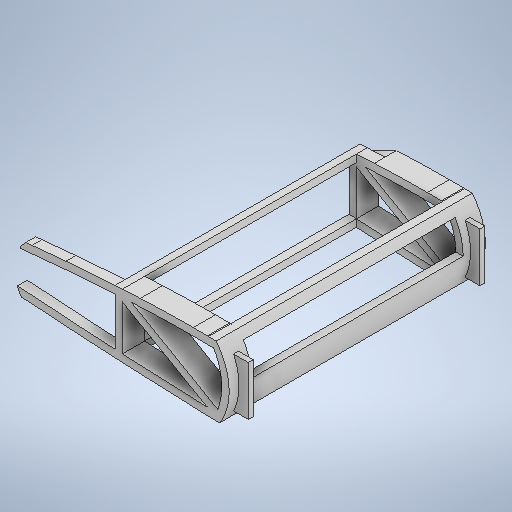
# Autodesk Inventor part: 1P.01.05.04-HB-PlatformFinala
Saved by Autodesk Inventor 2025.1 (Build 291241000, 241)
## iProperties
Created: 2025-01-16
Part Number: 1P.01.05.04-HB-PlatformFinala
Material: Generic
Document SubType Name: Modeling
Designer: hjbre
Density: 1 g/cm^3
Appearance: Default
Author: hjbre
Autodesk Inventor part; units mm, degrees
note: some values were not read from the file. Chosen so that the rebuilt part matches the saved one: second side of "Extrusion6".
ref_plane "YZ Plane" through (0, 0, 0) normal (1, 0, 0) x (0, 1, 0)
ref_plane "XZ Plane" through (0, 0, 0) normal (0, 1, 0) x (-1, 0, 0)
ref_plane "XY Plane" through (0, 0, 0) normal (0, 0, 1) x (1, 0, 0)
sketch "Sketch2" plane through (-116.745334, -43.168812, 0) normal (0, 0, 1) x (1, 0, 0)
  spline S0 degree 4 poles (254.436054, 38.258138) (252.159915, 38.650332) (246.788709, 39.499265) (237.984874, 40.618279) (225.357478, 41.704285) (211.202741, 42.341661) (196.392584, 42.47009) (181.031283, 42.070233) (165.506388, 41.221743) (149.785249, 40.04478) (134.1096, 38.577548) (118.624688, 36.850842) (103.500036, 34.939301) (88.901638, 32.883406) (74.995754, 30.738214) (61.917783, 28.562704) (49.827113, 26.40977) (38.835364, 24.340018) (29.07721, 22.403865) (20.632296, 20.65644) (13.645605, 19.149082) (6.913163, 17.660714) (2.90218, 16.740022) (0.469137, 16.188187) (0, 16.065) knots 0.21429705 0.21429705 0.21429705 0.21429705 0.21429705 0.2433201 0.28177524 0.32154178 0.36237973 0.40400459 0.44617789 0.48866482 0.5312306 0.57368816 0.61580317 0.65733642 0.6980466 0.73768213 0.77598623 0.81268845 0.84749504 0.88008735 0.91009265 0.93705903 0.9603631 1 1 1 1 1
  spline S1 degree 4 poles (299.999997, 15.624) (299.805651, 13.312974) (297.70854, 10.343184) (293.050897, 7.5008) (285.395888, 4.883043) (278.112378, 3.216454) (269.51472, 1.892454) (259.681019, 0.912997) (248.712883, 0.278332) (236.711867, -0.030891) (223.806667, -0.050368) (210.125319, 0.193333) (195.775416, 0.645033) (180.96771, 1.249367) (165.65166, 1.982539) (150.191633, 2.90484) (134.687258, 3.945111) (119.337536, 5.049498) (104.304233, 6.19869) (89.756609, 7.356132) (75.849243, 8.488651) (62.742937, 9.582405) (50.58108, 10.6226) (39.497058, 11.579661) (29.629443, 12.451258) (21.071102, 13.226419) (13.964229, 13.872003) (7.104281, 14.512735) (2.97189, 14.898983) (0.53364, 15.140199) (0, 15.183) knots 0 0 0 0 0 0.05437358 0.07982309 0.10791481 0.13850221 0.17134572 0.20619217 0.24278976 0.28089755 0.32028459 0.36072189 0.40203271 0.44399579 0.48638488 0.52897072 0.57147417 0.6136572 0.65528122 0.69610245 0.73587112 0.77432706 0.81119414 0.84617761 0.87895143 0.90913704 0.93627519 0.95973484 1 1 1 1 1
  arc A0 (0, 16.065) -> (0, 15.183) centre (0.115799, 15.624) ccw
  line L0 (0.115799, 15.624) -> (227.990221, 15.624) construction
  line L1 (299.999997, 15.624) -> (0.115799, 15.624) construction
  line L2 (299.999997, 15.624) -> (199.999997, 15.624) construction
  line L3 (199.999997, 15.624) -> (199.999997, 42.37734) construction
  line L4 (199.999997, 15.624) -> (199.999997, 0.52729)
  line L5 (0, 0) -> (0, 20.241)
  line L6 (0, 20.241) -> (238.581, 20.241) construction
  circle A1 centre (238.581, 20.241) radius 14
  line L7 (238.581, 20.241) -> (208.581, 20.241)
  line L8 (238.581, 25.359) -> (238.581, 20.241)
  line L9 (0, 20.241) -> (112, 20.241)
  circle A2 centre (112, 20.241) radius 5.39
  line L10 (0, 15.624) -> (112, 15.624) construction
  line L11 (0, 15.624) -> (112, 15.624) construction
  line L12 (112, 15.624) -> (112, 35.994456)
  line L13 (112, 15.624) -> (112, 5.61525)
  line L14 (299.207055, 20.082158) -> (298.87417, 19.536312) construction
  arc A3 (298.903999, 19.593162) -> (299.170168, 20.029611) centre (292.291091, 23.925437) ccw construction
  spline S2 degree 4 poles (299.285198, 20.241) (299.227939, 20.131643) (299.16804, 20.023225) (299.105573, 19.915754) (299.040612, 19.809235) knots 0 0 0 0 0 1 1 1 1 1
  line L15 (299.43203, 20.521431) -> (299.138367, 19.960569) construction
  arc A4 (299.163926, 20.01882) -> (299.398715, 20.467241) centre (292.801001, 23.636075) ccw construction
  line L16 (294.550692, 15.715716) -> (294.235931, 15.532284) construction
  arc A5 (294.267154, 15.551069) -> (294.518956, 15.69781) centre (283.884356, 33.65696) ccw construction
  spline S3 degree 2 poles (295.850621, 16.559978) (295.157262, 16.069203) (294.393311, 15.624) knots 0 0 0 1 1 1
  line L17 (295.959293, 16.465681) -> (295.74195, 16.654276) construction
  arc A6 (295.937354, 16.484307) -> (295.763482, 16.635181) centre (281.87292, 0.451609) ccw construction
  spline S4 degree 4 poles (296.856901, 15.624) (296.618326, 15.862944) (296.370731, 16.098547) (296.114674, 16.330852) (295.850621, 16.559978) knots 0 0 0 0 0 1 1 1 1 1
  spline S5 degree 4 poles (219.58717, 34.91187) (218.695351, 34.95198) (214.858509, 35.106335) (210.707211, 35.329502) (192.898023, 35.446366) (181.42777, 35.055508) (165.177387, 34.181901) (149.561876, 33.12667) (133.828431, 31.347909) (128.265438, 31.097419) (123.390775, 30.590026) knots 0 0 0 0 0 0.13924435 0.23321956 0.36393672 0.50998276 0.65711487 0.7981047 1 1 1 1 1
  line L18 (232.743774, 34.364452) -> (201.193566, 35.681454) construction
  arc A7 (229.586762, 34.454933) -> (204.347135, 35.508511) centre (136.348344, -1896.324468) ccw construction
  arc A8 (264.266057, 15.123) -> (264.360826, 15.624) centre (238.581, 20.241) ccw
  circle A9 centre (238.581, 20.241) radius 24
  circle A10 centre (112, 20.241) radius 15.39
  spline S6 degree 4 poles (299.999997, 15.624) (300.269142, 17.933652) (298.783415, 21.267693) (294.693448, 24.979847) (287.53174, 28.940551) (280.486947, 31.820538) (271.480983, 34.718213) (262.486804, 36.793013) (257.700386, 37.695672) (254.436054, 38.258138) knots 0 0 0 0 0 0.24755477 0.36385739 0.4925498 0.63299607 0.77826439 1 1 1 1 1
  line L19 (285.294543, 32.941011) -> (223.577565, 43.575266) construction
  arc A11 (278.722442, 32.634865) -> (229.668212, 41.087243) centre (217.218351, -177.738587) ccw construction
  line L20 (285.294543, 32.941011) -> (223.577565, 43.575266) construction
  arc A12 (278.877125, 33.041766) -> (229.658629, 41.522447) centre (200.894913, -272.473315) ccw construction
  line L21 (285.294543, 25.932171) -> (223.577565, 36.566425) construction
  spline S7 degree 4 poles (251.493, 31.73616) (243.700929, 32.967588) (232.160237, 34.296592) (216.442824, 35.287928) (196.392341, 35.461091) (181.031705, 35.061513) (165.505292, 34.212684) (149.788285, 33.036509) (134.101234, 31.567156) (118.647366, 29.846206) (103.439709, 27.919279) (89.058912, 25.903716) (74.837064, 23.692714) (62.488433, 21.669546) (49.639937, 19.354465) (46.379459, 18.742869) (43.812536, 18.259032) knots 0 0 0 0 0 0.1639631 0.23233838 0.3020312 0.37264227 0.44377843 0.51504665 0.58613365 0.65664712 0.72618654 0.7943479 0.86070997 0.92034602 1 1 1 1 1
  line L22 (285.294543, 25.932171) -> (223.577565, 36.566425) construction
  arc A13 (278.722442, 25.626025) -> (229.668212, 34.078402) centre (217.218351, -184.747428) ccw construction
  spline S8 degree 4 poles (295.845009, 16.556007) (295.719822, 16.664559) (294.584958, 17.628339) (292.058546, 19.428263) (287.516704, 21.93465) (280.467029, 24.832118) (271.97142, 27.522599) (264.208658, 29.400369) (258.409244, 30.551465) (255.053616, 31.142888) (254.436054, 31.249298) (253.968946, 31.329784) (253.501839, 31.41027) (253.034731, 31.490756) (252.567623, 31.571241) knots 0 0 0 0 0 0.01890503 0.16895946 0.33499927 0.51620401 0.71116085 0.9183366 0.96483207 0.96483207 0.96483207 0.96483207 1 1 1 1 1
  line L23 (270.129, 9.125374) -> (275.129, 9.125374) construction
  line L24 (281.07, 24.45816) -> (286.07, 24.45816) construction
  line L25 (318.821413, -3.367269) -> (272.868604, 36.479282) construction
  arc A14 (303.207925, 0.551953) -> (278.959518, 21.578206) centre (281.857648, 0.425162) ccw construction
  line L26 (68.488377, 16.119755) -> (19.136695, 20.398308) construction
  arc A15 (63.551474, 16.528056) -> (24.070206, 19.950891) centre (-819.899413, -9944.371227) ccw construction
  line L27 (21.724437, 20.217275) -> (21.200116, 20.264725) construction
  arc A16 (21.252548, 20.259982) -> (21.672005, 20.222022) centre (898.635849, 9712.955601) ccw construction
  spline S9 degree 4 poles (295.835285, 16.564433) (293.417091, 14.88464) (288.41352, 12.692641) (280.70627, 10.669821) (269.511023, 8.939829) (259.682627, 7.96324) (248.712204, 7.32734) (236.712148, 7.018633) (223.806545, 6.998947) (210.125394, 7.242728) (195.775305, 7.694406) (180.967993, 8.298721) (165.65086, 9.03198) (150.193891, 9.954022) (134.681006, 10.995018) (119.354518, 12.097424) (104.258979, 13.251926) (89.874814, 14.39542) (75.752353, 15.547068) (62.906491, 16.616479) (50.510696, 17.677636) (46.516568, 18.024605) (43.812536, 18.259032) knots 0 0 0 0 0 0.08476672 0.12402522 0.16617938 0.21090431 0.25787677 0.30678758 0.35734028 0.40924097 0.46226281 0.51612182 0.5705276 0.62518592 0.67973848 0.7338798 0.78730362 0.83969707 0.89073959 0.93714265 1 1 1 1 1
  spline S10 degree 4 poles (21.462276, 20.241) (20.622656, 20.316984) (20.124028, 20.362207) (19.919133, 20.380856) (19.554048, 20.414029) knots 0 0 0 0 0 1 1 1 1 1
  line L28 (74.254065, 23.996937) -> (13.371006, 12.521126) construction
  arc A17 (68.175943, 22.793945) -> (19.469999, 13.613391) centre (1053.390082, -5337.891027) ccw construction
  line L29 (133.533683, 10.96354) -> (115.839617, 12.094223) construction
  arc A18 (117.617989, 12.078874) -> (131.767822, 11.174674) centre (141.026952, 267.238396) ccw construction
  spline S11 degree 4 poles (218.437499, 7.193419) (217.617295, 7.240848) (213.819214, 7.468804) (209.586315, 6.850678) (192.548492, 7.944114) (181.146901, 8.16297) (165.746092, 9.02826) (149.142366, 9.880106) (139.977668, 10.751942) (129.107316, 11.246393) (124.68665, 11.528881) knots 0 0 0 0 0 0.12763083 0.21372336 0.33362841 0.4674456 0.60262129 0.73842442 0.88039529 0.88039529 0.88039529 0.88039529 0.88039529
  line L30 (140.664975, 32.388062) -> (106.116576, 28.79199) construction
  arc A19 (137.221962, 31.449676) -> (109.679039, 28.58279) centre (140.622493, -134.959578) ccw construction
  circle A20 centre (238.581, 20.241) radius 18
  line L31 (238.581, 38.241) -> (225.78, 41.559)
  line L32 (238.581, 2.241) -> (224.22, 0)
  line L33 (214.581, 20.241) -> (214.581, 42.126574) construction
  line L34 (127.39, 20.241) -> (127.39, 11.525517) construction
  line L35 (127.39, 20.241) -> (131.31394, 20.241) construction
  line L36 (96.61, 20.241) -> (96.61, 13.863077) construction
  line L37 (270.128995, 5.61525) -> (270.128995, 15.624) construction
  line L38 (272.128995, 7.61525) -> (272.128995, 13.624)
  line L39 (268.128995, 13.624) -> (268.128995, 7.61525)
  arc A21 (268.128995, 7.61525) -> (272.128995, 7.61525) centre (270.128995, 7.61525) ccw
  arc A22 (272.128995, 13.624) -> (268.128995, 13.624) centre (270.128995, 13.624) ccw
  line L40 (268.128995, 24.172) -> (268.128995, 30.18075)
  line L41 (270.128995, 32.18075) -> (270.128995, 22.172) construction
  arc A23 (272.128995, 30.18075) -> (268.128995, 30.18075) centre (270.128995, 30.18075) ccw
  line L42 (272.128995, 30.18075) -> (272.128995, 24.172)
  arc A24 (268.128995, 24.172) -> (272.128995, 24.172) centre (270.128995, 24.172) ccw
  arc A25 (199.999997, 42.315467) -> (199.853847, 42.377258) centre (190.581, 20.241) ccw
  arc A26 (171.272979, 34.495835) -> (171.268099, 34.489223) centre (190.581, 20.241) ccw
  arc A27 (210.748386, 7.230376) -> (209.287494, 35.276521) centre (190.581, 20.241) ccw
  arc A28 (169.445537, 8.870309) -> (169.474432, 8.816764) centre (190.581, 20.241) ccw
  arc A29 (153.976817, 9.682431) -> (154.030255, 9.739387) centre (142.78, 20.241) ccw
  arc A30 (151.241916, 33.095886) -> (151.219343, 33.110716) centre (142.78, 20.241) ccw
  arc A31 (132.12991, 31.350801) -> (130.322928, 11.203663) centre (142.78, 20.241) ccw
  arc A32 (95.274104, 13.969298) -> (95.169771, 26.74146) centre (81.22, 20.241) ccw
  arc A33 (66.333989, 16.334751) -> (66.538876, 15.624) centre (81.22, 20.241) ccw
  circle A34 centre (112, 20.241) radius 6.205
  circle A35 centre (238.581, 20.241) radius 15.15
  line L43 (209.287494, 35.276521) -> (209.287494, 7.228222) construction
  line L44 (209.287494, 35.276521) -> (237.335793, 35.276521) construction
  line L45 (270.128995, 22.172) -> (270.128995, 15.624) construction
  arc A36 (207.748386, 7.230376) -> (206.248584, 35.324804) centre (187.581, 20.241) ccw
  spline S12 degree 4 poles (211.366491, 32.239466) (210.846741, 32.24867) (210.326992, 32.257873) (209.807243, 32.267077) (209.287494, 32.27628) (209.049474, 32.280495) (208.811454, 32.28471) (208.573435, 32.288925) (208.335415, 32.293139) (207.212272, 32.313028) (202.665765, 32.376761) (191.8163, 32.412052) (181.353035, 32.055508) (165.102652, 31.181901) (149.487141, 30.12667) (133.753696, 28.347909) (128.190703, 28.097419) (123.31604, 27.590026) knots 0.15197941 0.15197941 0.15197941 0.15197941 0.15197941 0.17442836 0.17442836 0.17442836 0.17442836 0.18470888 0.18470888 0.18470888 0.18470888 0.23321956 0.36393672 0.50998276 0.65711487 0.7981047 1 1 1 1 1
  line L46 (215.794645, 32.161054) -> (200.876186, 32.425225) construction
  arc A37 (214.301175, 32.139448) -> (202.367955, 32.350757) centre (201.773375, -338.284165) ccw construction
  line L47 (133.515277, 13.96354) -> (115.821211, 15.094223) construction
  arc A38 (117.599583, 15.078874) -> (131.749417, 14.174674) centre (141.008546, 270.238396) ccw construction
  spline S13 degree 4 poles (209.384701, 10.211122) (207.978781, 10.200295) (203.438227, 10.242729) (192.03845, 10.953551) (181.128495, 11.16297) (165.727687, 12.02826) (149.12396, 12.880106) (139.959262, 13.751942) (129.08891, 14.246393) (124.668244, 14.528881) knots 0.1481124 0.1481124 0.1481124 0.1481124 0.1481124 0.21372336 0.33362841 0.4674456 0.60262129 0.73842442 0.88039529 0.88039529 0.88039529 0.88039529 0.88039529
  line L48 (216.905072, 10.269038) -> (201.864329, 10.153207) construction
  arc A39 (203.378671, 10.352301) -> (215.387843, 10.444785) centre (208.643229, 106.49222) ccw construction
  line L49 (168.289351, 34.321059) -> (168.289351, 8.879281)
  line L50 (171.268099, 34.489223) -> (171.268099, 8.723297)
  line L51 (172.446307, 33.103306) -> (211.548503, 10.663)
  line L52 (170.810346, 30.252646) -> (209.912542, 7.81234)
  line L53 (205.113566, 34.097762) -> (138.113825, 30.252646)
  line L54 (138.113825, 30.252646) -> (137.825505, 35.276521)
  line L55 (137.825505, 35.276521) -> (205.113566, 39.138185)
  line L56 (205.113566, 34.097762) -> (205.113566, 39.138185)
  line L57 (205.113566, 34.097762) -> (210.153989, 34.097762) construction
  line L58 (209.393078, 30.252646) -> (218.437499, 30.252646)
  line L59 (218.437499, 30.252646) -> (218.437499, 20.241)
  line L60 (218.437499, 10.229354) -> (218.437499, 20.241)
  line L61 (210.748386, 10.229354) -> (218.437499, 10.229354)
  line L62 (205.113566, 10.265254) -> (205.113566, 1.343815)
  line L63 (137.825505, 5.205479) -> (205.113566, 1.343815)
  line L64 (138.315622, 13.745588) -> (137.825505, 5.205479)
  line L65 (218.087064, 32.120461) -> (200.487923, 32.4321) construction
  arc A40 (202.247883, 32.403414) -> (216.327192, 32.154103) centre (386.335878, 10030.708851) ccw construction
  line L66 (127.39, 20.241) -> (125.098904, 20.241)
  line L67 (125.098904, 20.241) -> (125.098904, 30.18075)
  line L68 (125.098904, 30.18075) -> (127.39, 30.18075)
  line L69 (127.39, 30.18075) -> (127.39, 20.241)
  line L70 (127.39, 11.366827) -> (127.39, 20.241)
  line L71 (125.098904, 20.241) -> (125.098904, 11.502856)
  line L72 (215.794645, 29.161054) -> (200.876186, 29.425225) construction
  line L73 (218.087064, 29.120461) -> (200.487923, 29.4321) construction
  arc A41 (214.301175, 29.139448) -> (202.367955, 29.350757) centre (201.773375, -341.284165) ccw construction
  arc A42 (202.247883, 29.403414) -> (216.327192, 29.154103) centre (386.335878, 10027.708851) ccw construction
  spline S14 degree 4 poles (211.366491, 29.239466) (210.846741, 29.24867) (210.326992, 29.257873) (209.807243, 29.267077) (209.287494, 29.27628) (209.049474, 29.280495) (208.811454, 29.28471) (208.573435, 29.288925) (208.335415, 29.293139) (207.212272, 29.313028) (202.665765, 29.376761) (191.8163, 29.412052) (181.353035, 29.055508) (165.102652, 28.181901) (149.487141, 27.12667) (133.753696, 25.347909) (128.190703, 25.097419) (123.31604, 24.590026) knots 0.15197941 0.15197941 0.15197941 0.15197941 0.15197941 0.17442836 0.17442836 0.17442836 0.17442836 0.18470888 0.18470888 0.18470888 0.18470888 0.23321956 0.36393672 0.50998276 0.65711487 0.7981047 1 1 1 1 1
  line L74 (133.515277, 16.96354) -> (115.821211, 18.094223) construction
  line L75 (216.905072, 13.269038) -> (201.864329, 13.153207) construction
  arc A43 (117.599583, 18.078874) -> (131.749417, 17.174674) centre (141.008546, 273.238396) ccw construction
  arc A44 (203.378671, 13.352301) -> (215.387843, 13.444785) centre (208.643229, 109.49222) ccw construction
  spline S15 degree 4 poles (209.384701, 13.211122) (207.978781, 13.200295) (203.438227, 13.242729) (192.03845, 13.953551) (181.128495, 14.16297) (165.727687, 15.02826) (149.12396, 15.880106) (139.959262, 16.751942) (129.08891, 17.246393) (124.668244, 17.528881) knots 0.1481124 0.1481124 0.1481124 0.1481124 0.1481124 0.21372336 0.33362841 0.4674456 0.60262129 0.73842442 0.88039529 0.88039529 0.88039529 0.88039529 0.88039529
  line L76 (149.718265, 29.984) -> (149.718265, 26.984)
  line L77 (150.188594, 12.928) -> (150.188594, 15.928)
  line L78 (128.07267, 24.77383) -> (112, 26.446)
  line L79 (128.895582, 17.528881) -> (112, 14.036)
  line L80 (135.213001, 15.013) -> (136.481046, 8.879281)
  line L81 (135.213001, 25.469) -> (137.991389, 38.908473)
  line L82 (112, 25.210875) -> (94.804772, 25.210875)
  line L83 (94.804772, 25.210875) -> (94.804772, 15.210875)
  line L84 (94.804772, 15.210875) -> (112, 15.210875)
  line L85 (112, 15.210875) -> (112, 25.210875)
  line L86 (230.468449, 4.172817) -> (136.481046, 8.879281)
  line L87 (230.468449, 4.172817) -> (230.468449, 36.309183)
  line L88 (137.454029, 36.309183) -> (128.07267, 29.984)
  line L89 (136.481046, 8.879281) -> (127.39, 11.525517)
  line L90 (230.468449, 36.309183) -> (230.468449, 38.073091)
  line L91 (230.468449, 38.073091) -> (137.454029, 36.309183)
  point P0 (0.783, 16.254)
  point P1 (3.213, 16.812)
  point P2 (7.239, 17.724)
  point P3 (12.813, 18.96)
  point P4 (19.884, 20.484)
  point P5 (28.374, 22.245)
  point P6 (38.199, 24.195)
  point P7 (49.254, 26.28)
  point P8 (61.419, 28.446)
  point P9 (74.571, 30.636)
  point P10 (88.56, 32.793)
  point P11 (103.242, 34.86)
  point P12 (118.455, 36.783)
  point P13 (134.028, 38.511)
  point P14 (149.793, 39.984)
  point P15 (165.576, 41.16)
  point P16 (181.206, 41.985)
  point P17 (196.638, 42.363)
  point P18 (211.554, 42.222)
  point P19 (239.145, 40.389)
  point P20 (262.68, 36.666)
  point P21 (272.577, 34.218)
  point P22 (281.07, 31.467)
  point P23 (288.069, 28.491)
  point P24 (293.505, 25.359)
  point P25 (297.324, 22.137)
  point P26 (300, 15.624)
  point P27 (0.861, 15.105)
  point P28 (3.342, 14.868)
  point P29 (7.446, 14.481)
  point P30 (13.122, 13.953)
  point P31 (20.31, 13.296)
  point P32 (28.92, 12.519)
  point P33 (38.856, 11.64)
  point P34 (50.007, 10.674)
  point P35 (62.244, 9.63)
  point P36 (75.429, 8.529)
  point P37 (89.418, 7.389)
  point P38 (104.052, 6.228)
  point P39 (119.172, 5.076)
  point P40 (134.613, 3.966)
  point P41 (150.207, 2.928)
  point P42 (165.783, 2.013)
  point P43 (181.167, 1.263)
  point P44 (196.068, 0.663)
  point P45 (210.468, 0.225)
  point P46 (237.189, 0.039)
  point P47 (249.246, 0.378)
  point P48 (260.262, 1.05)
  point P49 (270.129, 2.076)
  point P50 (278.739, 3.462)
  point P51 (285.993, 5.211)
  point P52 (291.81, 7.314)
  point P53 (296.121, 9.756)
  point P54 (298.863, 12.531)
  point P55 (199.999997, 15.624)
  point P56 (225.364219, 15.624)
  point P57 (238.581, 6.241)
  point P58 (238.581, 34.241)
  point P59 (225.364219, 15.624)
  point P60 (251.797781, 15.624)
  point P61 (0, 16.065)
  point P62 (0, 15.183)
  point P63 (224.581, 20.241)
  point P64 (112, 14.851)
  point P65 (112, 25.631)
  point P66 (0, 9.065)
  point P67 (0.783, 9.254)
  point P68 (3.213, 9.812)
  point P69 (7.239, 10.724)
  point P70 (12.813, 11.96)
  point P71 (19.884, 13.484)
  point P72 (28.374, 15.245)
  point P73 (38.199, 17.195)
  point P74 (49.254, 19.28)
  point P75 (61.419, 21.446)
  point P76 (74.571, 23.636)
  point P77 (88.56, 25.793)
  point P78 (103.242, 27.86)
  point P79 (118.455, 29.783)
  point P80 (134.028, 31.511)
  point P81 (149.793, 32.984)
  point P82 (165.576, 34.16)
  point P83 (181.206, 34.985)
  point P84 (225.78, 34.559)
  point P85 (239.145, 33.389)
  point P86 (251.493, 31.745)
  point P87 (262.68, 29.666)
  point P88 (272.577, 27.218)
  point P89 (281.07, 24.467)
  point P90 (288.069, 21.491)
  point P91 (293.505, 18.359)
  point P92 (297.324, 15.137)
  point P93 (299.493, 11.879)
  point P94 (300, 8.624)
  point P95 (-0.004161, 22.184114)
  point P96 (0.861, 22.105)
  point P97 (3.342, 21.868)
  point P98 (7.446, 21.481)
  point P99 (13.122, 20.953)
  point P100 (20.31, 20.296)
  point P101 (28.92, 19.519)
  point P102 (38.856, 18.64)
  point P103 (50.007, 17.674)
  point P104 (62.244, 16.63)
  point P105 (75.429, 15.529)
  point P106 (89.418, 14.389)
  point P107 (104.052, 13.228)
  point P108 (119.172, 12.076)
  point P109 (134.613, 10.966)
  point P110 (150.207, 9.928)
  point P111 (165.783, 9.013)
  point P112 (181.167, 8.263)
  point P113 (196.068, 7.663)
  point P114 (210.468, 7.225)
  point P115 (224.22, 7)
  point P116 (237.189, 7.039)
  point P117 (249.246, 7.378)
  point P118 (260.262, 8.05)
  point P119 (270.129, 9.076)
  point P120 (278.739, 10.462)
  point P121 (285.993, 12.211)
  point P122 (291.81, 14.314)
  point P123 (296.121, 16.756)
  point P124 (298.863, 19.531)
  point P125 (300, 22.624)
  point P126 (18.740477, 20.241)
  point P127 (216.96867, 35.022953)
  point P128 (0, 16.065)
  point P129 (296.856901, 15.624)
  point P130 (294.393311, 15.624)
  point P131 (219.58717, 34.91187)
  point P132 (123.390775, 30.590026)
  point P133 (254.436054, 38.258138)
  point P134 (0, 9.05616)
  point P135 (0.783, 9.24516)
  point P136 (3.213, 9.80316)
  point P137 (7.239, 10.71516)
  point P138 (12.813, 11.95116)
  point P139 (19.884, 13.47516)
  point P140 (28.374, 15.23616)
  point P141 (38.199, 17.18616)
  point P142 (49.254, 19.27116)
  point P143 (61.419, 21.43716)
  point P144 (74.571, 23.62716)
  point P145 (88.56, 25.78416)
  point P146 (103.242, 27.85116)
  point P147 (118.455, 29.77416)
  point P148 (134.028, 31.50216)
  point P149 (149.793, 32.97516)
  point P150 (165.576, 34.15116)
  point P151 (181.206, 34.97616)
  point P152 (196.638, 35.35416)
  point P153 (211.554, 35.21316)
  point P154 (225.78, 34.55016)
  point P155 (254.436054, 31.249298)
  point P156 (278.876889, 26.073396)
  point P157 (229.590604, 33.866167)
  point P158 (216.884838, -206.362485)
  point P159 (262.68, 29.65716)
  point P160 (272.577, 27.20916)
  point P161 (297.324, 15.12816)
  point P162 (299.493, 11.87016)
  point P163 (300, 8.61516)
  point P164 (-0.004161, 22.233488)
  point P165 (0.861, 22.154374)
  point P166 (3.342, 21.917374)
  point P167 (7.446, 21.530374)
  point P168 (13.122, 21.002374)
  point P169 (28.92, 19.568374)
  point P170 (38.856, 18.689374)
  point P171 (50.007, 17.723374)
  point P172 (62.244, 16.679374)
  point P173 (75.429, 15.578374)
  point P174 (89.418, 14.438374)
  point P175 (104.052, 13.277374)
  point P176 (119.172, 12.125374)
  point P177 (134.613, 11.015374)
  point P178 (150.207, 9.977374)
  point P179 (165.783, 9.062374)
  point P180 (181.167, 8.312374)
  point P181 (196.068, 7.712374)
  point P182 (210.468, 7.274374)
  point P183 (224.22, 7.049374)
  point P184 (237.189, 7.088374)
  point P185 (249.246, 7.427374)
  point P186 (260.262, 8.099374)
  point P187 (278.739, 10.511374)
  point P188 (285.993, 12.260374)
  point P189 (296.121, 16.805374)
  point P190 (298.863, 19.580374)
  point P191 (300, 22.673374)
  point P192 (225.700031, -0.009448)
  point P193 (252.261653, 0.521981)
  point P194 (227.349521, 41.450759)
  point P195 (105.977751, 6.07821)
  point P196 (115.800844, 5.327728)
  point P197 (98.259993, 27.173842)
  point P198 (260.452219, 30.122789)
  point P199 (123.585295, 30.371797)
  dimension "d56" = 100
  dimension "d55" = 20.241
  dimension "d54" = 238.581
  dimension "d53" = 28
  dimension "d52" = 112
  dimension "d51" = 10.78
  dimension "d50" = 112
  dimension "d69" = 0
  dimension "d48" = 10
  dimension "d47" = 10
  dimension "d43" = 4
  dimension "d70" = 90
  dimension "d42" = 4
  dimension "d41" = 12.41
  dimension "d40" = 30.3
  dimension "d39" = 90
  dimension "d38" = 209.62764
  dimension "d37" = 270.46915
  dimension "d46" = 7.00884
  dimension "d44" = 7.04937
  dimension "d49" = 7
  dimension "d45" = 7.04937
  dimension "d36" = 6.548
  dimension "d35" = 90
  constraints: 187 end point, 83 point on circle, 48 midpoint, 45 centre point, 31 point on line, 14 perpendicular, 13 symmetric about line, 12 horizontal, 7 parallel, 7 tangent, 4 coincident, 3 collinear, 3 equal length, 3 vertical, 260 other
  measures "d56" distance of L1.start L2.end
  measures "d55" distance of L5.start L5.end
  measures "d54" distance of L5.end L6.end
  measures "d53" diameter of A1
  measures "d52" distance of L5.end L9.end
  measures "d51" diameter of A2
  measures "d50" distance of L10.start L10.end
  measures "d69" distance between parallel lines of L11 L10
  measures "d48" radial gap between concentric circles of A1 A9
  measures "d47" radial gap between concentric circles of A2 A10
  measures "d43" radial gap between concentric circles of A1 A20
  measures "d70" angle of L34 L35
  measures "d42" diameter of A22
  measures "d41" diameter of A34
  measures "d40" diameter of A35
  measures "d39" angle of L43 L44
  measures "d38" distance from line of point (-0.34, 15.624) L43
  measures "d37" horizontal distance of point (-0.34, 15.624) point (270.129, 18.898)
  measures "d46" distance of point (196.638, 35.354) point (196.638, 42.363)
  measures "d44" distance of point (196.068, 0.663) point (196.068, 7.712)
  measures "d49" distance of point (149.793, 32.984) point (149.793, 39.984)
  measures "d45" distance of point (150.207, 2.928) point (150.207, 9.977)
  measures "d36" distance of point (270.129, 15.624) point (270.129, 22.172)
  measures "d35" angle of L57 L56
extrude "Extrusion3" add sketch "Sketch2" along normal blind 4 and the other way blind 48 contours S5 A27 S7 | S7 A27 S12 A36 | A27 S9 A36 L7 | L50 L53 L49 S5 | S5 S7 A26 | L50 S12 L49 L53 | S13 L50 S9 L49 picked at (208.277757, 35.288881) picked at (170.275725, 34.433903)
sketch "Sketch2 outline for Extrusion4" plane through (-116.745334, -43.168812, 0) normal (0, 0, 1) x (1, 0, 0)
  spline S0 degree 4 poles (148.35454, 32.852821) (146.835905, 32.712718) (143.210993, 32.368194) (139.588936, 32.009223) (136.35466, 31.713592) (134.59788, 31.560388) knots 0 0 0 0 0 0.42221913 1 1 1 1 1
  spline S1 degree 4 poles (168.289351, 34.321059) (165.638345, 34.160064) (160.661405, 33.832977) (155.672123, 33.463029) (150.682324, 33.052791) (148.35454, 32.852821) knots 0 0 0 0 0 0.5332904 1 1 1 1 1
  line L0 (168.289351, 31.325383) -> (168.289351, 34.321059)
  spline S2 degree 4 poles (168.289351, 31.325383) (165.597326, 31.169704) (159.176149, 30.774834) (149.790951, 30.088629) (138.279154, 28.847823) (132.329062, 28.371598) (129.576995, 28.148765) knots 0 0 0 0 0 0.2697022 0.64939644 1 1 1 1 1
  arc A0 (132.077253, 31.300083) -> (129.576995, 28.148765) centre (142.78, 20.241) ccw
  spline S3 degree 4 poles (134.59788, 31.560388) (133.967323, 31.496162) (133.337031, 31.431366) (132.707007, 31.366004) (132.077253, 31.300083) knots 0 0 0 0 0 1 1 1 1 1
  spline S4 degree 4 poles (210.748386, 7.230376) (209.158857, 7.198173) (204.646728, 7.167636) (192.453603, 7.945936) (181.146901, 8.16297) (165.746092, 9.02826) (150.424265, 9.814339) (141.886646, 10.576084) (133.759076, 11.015279) (130.322928, 11.203663) knots 0 0 0 0 0 0.11624636 0.28593982 0.47532218 0.66662714 0.85882006 1 1 1 1 1
  arc A1 (128.58353, 14.298582) -> (130.322928, 11.203663) centre (142.78, 20.241) ccw
  spline S5 degree 4 poles (168.289351, 11.878306) (165.651133, 12.018029) (158.943337, 12.381198) (148.989661, 12.928043) (141.294499, 13.627761) (132.420781, 14.084935) (128.58353, 14.298582) knots 0 0 0 0 0 0.26556409 0.66759842 1 1 1 1 1
  line L1 (168.289351, 31.325383) -> (168.289351, 11.878306)
  spline S6 degree 4 poles (171.268099, 31.493335) (170.522352, 31.452333) (169.776533, 31.410643) (169.031982, 31.36833) (168.289351, 31.325383) knots 0 0 0 0 0 1 1 1 1 1
  line L2 (171.268099, 34.489223) -> (171.268099, 31.493335)
  spline S7 degree 4 poles (178.528633, 34.863187) (177.276364, 34.803751) (175.47804, 34.714424) (173.646614, 34.618937) (171.809328, 34.519018) (171.268099, 34.489223) knots 0 0 0 0 0 0.70542122 1 1 1 1 1
  spline S8 degree 4 poles (200.033241, 35.36854) (197.255545, 35.367651) (191.907201, 35.320018) (186.514748, 35.186583) (181.112865, 34.978379) (178.528633, 34.863187) knots 0 0 0 0 0 0.52193064 1 1 1 1 1
  spline S9 degree 4 poles (205.775807, 35.331387) (205.189474, 35.338212) (203.813251, 35.352153) (202.354101, 35.362146) (200.86779, 35.36729) (200.033241, 35.36854) knots 0 0 0 0 0 0.43964902 1 1 1 1 1
  spline S10 degree 4 poles (206.248584, 35.324804) (206.130431, 35.326517) (206.01225, 35.328185) (205.894042, 35.329809) (205.775807, 35.331387) knots 0 0 0 0 0 1 1 1 1 1
  arc A2 (208.335415, 32.293139) -> (206.248584, 35.324804) centre (187.581, 20.241) ccw
  spline S11 degree 4 poles (208.335415, 32.293139) (207.212272, 32.313028) (202.665765, 32.376761) (192.300341, 32.410478) (185.261946, 32.187901) (178.42894, 31.868771) (174.913227, 31.687568) knots 0 0 0 0 0 0.15610236 0.57673667 1 1 1 1 1
  line L3 (209.961354, 11.573847) -> (174.913227, 31.687568)
  arc A3 (207.819833, 7.341797) -> (209.961354, 11.573847) centre (187.581, 20.241) ccw
  spline S12 degree 4 poles (210.772011, 7.267069) (210.035733, 7.28465) (209.29825, 7.302982) (208.559601, 7.32204) (207.819833, 7.341797) knots 0 0 0 0 0 1 1 1 1 1
  arc A4 (210.748386, 7.230376) -> (210.772011, 7.267069) centre (190.581193, 20.240876) ccw
  line L4 (168.289351, 8.929952) -> (168.289351, 11.878306)
  spline S13 degree 4 poles (171.268099, 8.7781) (170.523996, 8.815301) (169.779456, 8.853004) (169.034554, 8.891219) (168.289351, 8.929952) knots 0 0 0 0 0 1 1 1 1 1
  line L5 (171.268099, 11.722347) -> (171.268099, 8.7781)
  spline S14 degree 4 poles (171.268099, 11.722347) (170.528788, 11.760518) (169.785346, 11.79933) (169.038561, 11.838627) (168.289351, 11.878306) knots 0 0 0 0 0 1 1 1 1 1
  spline S15 degree 4 poles (205.665234, 10.249822) (204.926632, 10.269121) (200.754913, 10.405277) (191.118223, 10.971215) (183.893246, 11.1099) (176.292704, 11.464956) (171.848414, 11.692385) (171.268099, 11.722347) knots 0 0 0 0 0 0.09061443 0.48897983 0.93356606 1 1 1 1 1
  line L6 (171.268099, 29.989946) -> (205.665234, 10.249822)
  line L7 (171.268099, 11.722347) -> (171.268099, 29.989946)
  arc A5 (214.580996, 20.241) -> (211.366491, 32.239466) centre (190.581, 20.241) ccw
  line L8 (211.580996, 20.241) -> (214.580996, 20.241)
  arc A6 (208.335415, 32.293139) -> (211.580996, 20.241) centre (187.581, 20.241) cw
  spline S16 degree 4 poles (211.366491, 32.239466) (210.846741, 32.24867) (210.326992, 32.257873) (209.807243, 32.267077) (209.287494, 32.27628) (209.049474, 32.280495) (208.811454, 32.28471) (208.573435, 32.288925) (208.335415, 32.293139) knots 0 0 0 0 0 0.68589415 0.68589415 0.68589415 0.68589415 1 1 1 1 1
extrude "Extrusion4" add sketch "Sketch2 outline for Extrusion4" along normal blind 4 and the other way blind 5
extrude "Extrusion5" add sketch "Sketch2" against normal blind 2 contours L58 L59 L7 A9 | A9 A27 L58 | L7 L60 L61 A9 | A9 L61 A27
mirror "Mirror2" about plane through (94.45508, -29.414778, -48) normal (0, 0, -1) of "Extrusion3", "Extrusion4", "Extrusion5"
sketch "Sketch2 outline for Extrusion6" plane through (-116.745334, -43.168812, 0) normal (0, 0, 1) x (1, 0, 0)
  spline S0 degree 4 poles (148.35454, 32.852821) (146.835905, 32.712718) (143.210993, 32.368194) (139.588936, 32.009223) (136.35466, 31.713592) (134.59788, 31.560388) knots 0 0 0 0 0 0.42221913 1 1 1 1 1
  spline S1 degree 4 poles (168.289351, 34.321059) (165.638345, 34.160064) (160.661405, 33.832977) (155.672123, 33.463029) (150.682324, 33.052791) (148.35454, 32.852821) knots 0 0 0 0 0 0.5332904 1 1 1 1 1
  line L0 (168.289351, 31.325383) -> (168.289351, 34.321059)
  spline S2 degree 4 poles (168.289351, 31.325383) (165.597326, 31.169704) (159.176149, 30.774834) (149.790951, 30.088629) (138.279154, 28.847823) (132.329062, 28.371598) (129.576995, 28.148765) knots 0 0 0 0 0 0.2697022 0.64939644 1 1 1 1 1
  arc A0 (132.077253, 31.300083) -> (129.576995, 28.148765) centre (142.78, 20.241) ccw
  spline S3 degree 4 poles (134.59788, 31.560388) (133.967323, 31.496162) (133.337031, 31.431366) (132.707007, 31.366004) (132.077253, 31.300083) knots 0 0 0 0 0 1 1 1 1 1
  spline S4 degree 4 poles (168.289351, 8.879281) (165.655578, 9.018785) (158.952523, 9.381704) (149.373522, 9.908089) (141.886646, 10.576084) (133.759076, 11.015279) (130.322928, 11.203663) knots 0 0 0 0 0 0.27544119 0.69315689 1 1 1 1 1
  arc A1 (128.58353, 14.298582) -> (130.322928, 11.203663) centre (142.78, 20.241) ccw
  spline S5 degree 4 poles (168.289351, 11.878306) (165.651133, 12.018029) (158.943337, 12.381198) (148.989661, 12.928043) (141.294499, 13.627761) (132.420781, 14.084935) (128.58353, 14.298582) knots 0 0 0 0 0 0.26556409 0.66759842 1 1 1 1 1
  line L1 (168.289351, 8.879281) -> (168.289351, 11.878306)
extrude "Extrusion6" cut sketch "Sketch2 outline for Extrusion6" against normal blind 120
sketch "Sketch3" plane through (51.544016, -34.289531, -100) normal (0, 0, -1) x (-1, 0, 0)
  ellipse E0 centre (-2.936297, 25.404836) end of major axis (-17.851909, 26.226581) minor radius 0.202462 (-2.978749, 25.609942) -> (-10.239283, 25.983906) ccw
  line L0 (-10.239283, 25.983906) -> (0, 20.918287)
  line L1 (0, 0) -> (0, 25.441778)
  line L2 (0, 25.441778) -> (0, 20.918287)
  line L3 (-10.239283, 25.983906) -> (0, 25.441778)
  line L4 (-10.239283, 25.983906) -> (-10.239283, 26.254337)
  line L5 (-2.963902, 25.879661) -> (0, 25.441778)
  spline S0 degree 3 poles (-2.963906, 25.879588) (-5.388582, 26.013038) (-7.813669, 26.13918) (-10.239287, 26.254254) knots 0 0 0 0 1 1 1 1
  point P0 (51.544016, 34.289531)
  constraints: 10 end point, 1 collinear, 1 point on line, 1 vertical, 4 other
extrude "Extrusion7" cut sketch "Sketch3" against normal blind 4.6
body "Solid2"
